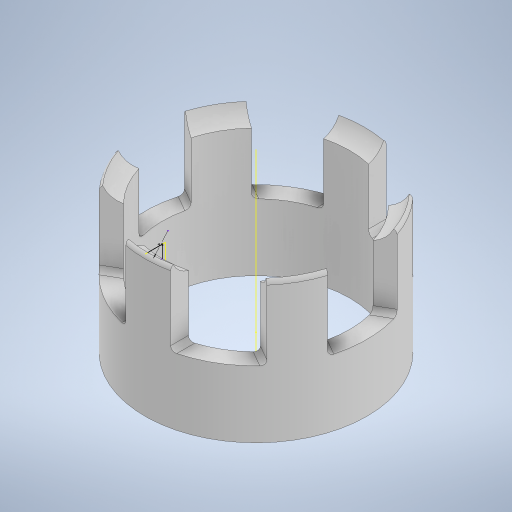
# Autodesk Inventor part: 다단로켓벨브2_ver3
Saved by Autodesk Inventor 2023 (Build 270158000, 158)
## iProperties
Created: 2023-08-25
Part Number: 다단로켓벨브2_ver3
Material: 일반
Document SubType Name: Modeling
Designer: rlatk
Density: 1 g/cm^3
Appearance: 기본값
Author: rlatk
Autodesk Inventor part; units mm, degrees
ref_plane "YZ Plane" through (0, 0, 0) normal (1, 0, 0) x (0, 1, 0)
ref_plane "XZ Plane" through (0, 0, 0) normal (0, 1, 0) x (-1, 0, 0)
ref_plane "XY Plane" through (0, 0, 0) normal (0, 0, 1) x (1, 0, 0)
sketch "스케치1" plane through (0, 0, 0) normal (0, 1, 0) x (-1, 0, 0)
  circle A0 centre (0, 0) radius 19
  circle A1 centre (0, 0) radius 22.5
  dimension "d0" = 38
  dimension "d1" = 3.5
  constraints: 2 centre point, 1 coincident
  measures "d0" diameter of A0
  measures "d1" radial gap between concentric circles of A0 A1
extrude "돌출1" add sketch "스케치1" along normal blind 10
sketch "스케치2" plane through (0, 10, 0) normal (0, 1, 0) x (1, 0, 0)
  line L0 (-4.2948, -18.7329) -> (-4.2948, -22.0863)
  line L1 (-3.2948, 22.2575) -> (-3.2948, 20.2507)
  circle A0 centre (0, 0) radius 22.5 projected
  circle A1 centre (0, 0) radius 19 projected
  line L2 (-4.2948, -22.0863) -> (-4.2948, -18.5082)
  line L3 (-3.2948, 18.7121) -> (-3.2948, 22.2575)
  line L4 (4.7052, -22.0025) -> (4.7052, -18.4082)
  line L5 (3.2948, 18.7121) -> (3.2948, 22.2575)
  arc A2 (-1.7487, -22.4319) -> (4.7052, -22.0025) centre (0, 0) ccw
  arc A3 (3.2948, 22.2575) -> (-1.7487, 22.4319) centre (0, 0) ccw
  arc A4 (-1.6474, -18.9284) -> (4.7052, -18.4082) centre (0, 0) ccw
  arc A5 (3.2948, 18.7121) -> (-1.6474, 18.9284) centre (0, 0) ccw
  arc A6 (-4.2948, -22.0863) -> (4.7052, -22.0025) centre (0, 0) ccw
  arc A7 (3.2948, 22.2575) -> (-3.2948, 22.2575) centre (0, 0) ccw
  arc A8 (-4.2948, -18.5082) -> (4.7052, -18.4082) centre (0, 0) ccw
  arc A9 (3.2948, 18.7121) -> (-3.2948, 18.7121) centre (0, 0) ccw
  point P0 (-3, 19.0654)
  point P1 (-1.5, 17.2348)
  point P2 (-1.5, -17.2348)
  point P3 (-3, -19.0654)
  point P4 (4.7052, -18.4082)
  point P5 (-1.7487, 22.4319)
  point P6 (3.2948, 22.2575)
  point P7 (-1.6474, -18.9284)
  point P8 (4.7052, -18.4082)
  dimension "d42" = 9
  constraints: 20 point on circle, 12 end point, 8 centre point, 5 vertical, 4 coincident
  measures "d42" distance between parallel lines of L4 L0
extrude "돌출4" add sketch "스케치2" along normal blind 15 contours L2 A1 L4 A0 L0
sketch "스케치7" plane through (0, 0, 0) normal (1, 0, 0) x (0, 1, 0)
  line L0 (25, 22.0863) -> (25, 22.5) projected
  line L1 (25, 19) -> (25, 18.4082) projected
  line L2 (25, 18.4082) -> (25, 22.0863) projected
  line L3 (25, 19) -> (0, 19) projected
  arc A0 (25, 21.9939) -> (22.4115, 19) centre (26.763, 17.8537) ccw
  line L4 (25, 21.9939) -> (25, 19)
  line L5 (25, 19) -> (22.4115, 19)
  line L6 (10, 18.5082) -> (25, 18.5082) projected
  line L7 (-5.3526, 0) -> (32.1156, 0) projected
  point P0 (0, 0)
  dimension "d32" = 4.5
  constraints: 4 end point, 2 point on circle, 2 point on line, 1 centre point, 1 collinear, 1 parallel
  measures "d32" radius of A0
revolve "회전3" cut sketch "스케치7" angle 360 about axis through (0, -10, 0) along (0, 1, 0)
pattern_circular "원형 패턴3" count 6 over 360 about axis through (0, -10, 0) along (0, 1, 0) of "돌출4"
revolve "회전4" cut sketch "스케치7" angle 360 about axis through (0, -10, 0) along (0, -1, 0)
fillet "모깎기4" radius 1 23 edges at (15.1457, 10, -14.1775) (18.2733, 10, -5.5909) (19.8226, 10, -6.4854) (-4.7052, 10, -20.2054) (4.2948, 10, -18.6206) (4.2948, 10, -20.4096) (-13.9785, 10, -13.0297) (-15.5278, 10, -13.9242) (-19.8509, 10, -6.0279) (-18.2733, 10, 5.5909) (-19.8226, 10, 6.4854) (-15.1457, 10, 14.1775) (-4.2948, 10, 20.2973) (4.7052, 10, 20.2054) (13.9785, 10, 13.0297) (15.5278, 10, 13.9242) (19.8509, 10, 6.0279) (19.5894, 25, 11.0681) (0.2094, 25, 22.499) (-19.38, 25, 11.4309) (-19.5894, 25, -11.0681) (-0.2094, 25, -22.499) (19.38, 25, -11.4309)
sketch "스케치8" plane through (0, 0, 0) normal (0, -1, 0) x (1, 0, 0)
  point P0 (0, 0)
sketch "스케치9" plane through (0, 0, 0) normal (0, -1, 0) x (1, 0, 0)
  circle A0 centre (0, 0) radius 22.5 projected
  circle A1 centre (0, 0) radius 19 projected
  circle A2 centre (0, 0) radius 22.5
  circle A3 centre (0, 0) radius 19
  constraints: 2 centre point, 2 coincident, 1 concentric
extrude "돌출5" add sketch "스케치9" along normal blind 3.5
